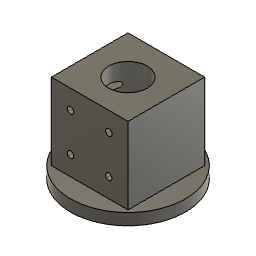
splicer_sample-fixation_016 (Autodesk Fusion 360 design; units mm, degrees)
Autodesk Fusion 360 part; units mm, degrees
sketch "Sketch1" plane through (0, 0, 0) normal (0, 1, 0) x (1, 0, 0)
  line L0 (47.5, -22.5) -> (-47.5, -22.5)
  line L1 (-47.5, -22.5) -> (-47.5, 22.5)
  line L2 (-47.5, 22.5) -> (47.5, 22.5)
  line L3 (47.5, 22.5) -> (47.5, -22.5)
  line L4 (47.5, -22.5) -> (-47.5, 22.5) construction
  line L5 (-47.5, -22.5) -> (47.5, 22.5) construction
  line L6 (20, -20) -> (-20, -20)
  line L7 (-20, -20) -> (-20, 20)
  line L8 (-20, 20) -> (20, 20)
  line L9 (20, 20) -> (20, -20)
  line L10 (20, -20) -> (-20, 20) construction
  line L11 (-20, -20) -> (20, 20) construction
  circle A0 centre (0, 0) radius 30
  point P0 (-41, 0)
  point P1 (41, 0)
  dimension "d1" = 95
  dimension "d2" = 45
  dimension "d3" = 82
  dimension "d4" = 41
  dimension "d11" = 40
  dimension "d12" = 40
  dimension "d26" = 60
  constraint horizontal L0
  constraint perpendicular L0 L1
  constraint parallel L0 L2
  constraint parallel L1 L3
  constraint coincident L4 A0.centre
  constraint coincident L5 A0.centre
  constraint coincident A0.centre origin
  constraint horizontal L6
  constraint perpendicular L6 L7
  constraint parallel L6 L8
  constraint parallel L7 L9
  constraint coincident L10 A0.centre
  constraint coincident L11 A0.centre
  measures "d1" distance of L1.end L2.end
  measures "d2" distance of L0.end L1.end
  measures "d3" distance of P0 P1
  measures "d4" distance of A0.centre P0
  measures "d11" distance of L7.end L8.end
  measures "d12" distance of L6.end L7.end
  measures "d26" diameter of A0
extrude "Extrude1" add sketch "Sketch1" against normal blind 6 contours L0 A0 | L0 L2 A0 | L2 A0 | L6 L7 L8 L9
hole "Hole1" at (-41, 0, 0) at (41, 0, 0) direction (0, -1, 0) diameter 3.4 depth 35 tip angle 118 counterbore diameter 6.5 counterbore depth 3
extrude "Extrude2" add sketch "Sketch1" along normal blind 40 contours L6 L7 L8 L9
sketch "Sketch2" plane through (0, 0, 20) normal (0, 0, 1) x (1, 0, 0)
  line L0 (-20, 0) -> (20, 0)
  line L1 (20, 0) -> (20, 40)
  line L2 (20, 40) -> (-20, 40)
  line L3 (-20, 40) -> (-20, 0)
  point P0 (-10, 30)
  point P1 (10, 30)
  point P2 (10, 10)
  point P3 (-10, 10)
hole "Hole2" at (10, 30, 20) at (-10, 30, 20) at (-10, 10, 20) at (10, 10, 20) direction (0, 0, -1) diameter 3.4 depth 44 tip angle 118
sketch "Sketch3" plane through (0, 40, 0) normal (0, 1, 0) x (-1, 0, 0)
  line L0 (-20, -20) -> (20, -20)
  line L1 (20, -20) -> (20, 20)
  line L2 (20, 20) -> (-20, 20)
  line L3 (-20, 20) -> (-20, -20)
hole "Hole3" at (0, 40, 0) direction (0, -1, 0) diameter 3.5 depth 50 tip angle 118 counterbore diameter 20 counterbore depth 38
equation "d4 = d3 / 2"
named bodies: "splicer-fixation_centerpoint"
